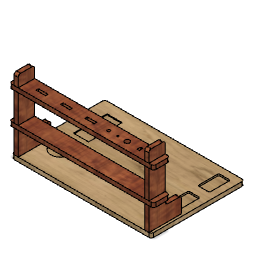
Soldering deskk 18mm v4 (Autodesk Fusion 360 design; units mm, degrees)
Autodesk Fusion 360 part; units mm, degrees
sketch "Limits" plane through (0, 0, 0) normal (0, 1, 0) x (1, 0, 0) in component "Soldering desk v11"
  line L0 (0, 0) -> (-1200, 0)
  line L1 (-1200, 0) -> (-1200, -1200)
  line L2 (-1200, -1200) -> (0, -1200)
  line L3 (0, -1200) -> (0, 0)
  dimension "d5" = 1200
  dimension "d6" = 1200
  constraint horizontal L0
  constraint vertical L1
  constraint horizontal L2
  constraint vertical L3
  constraint coincident L0.start L3.end
  measures "d5" distance of L0.start L0.end
  measures "d6" distance of L0.start L2.end
sketch "Soldering Base" plane through (0, 0, 0) normal (0, 1, 0) x (1, 0, 0) in component "Soldering desk v11"
  line L0 (0, 0) -> (-600, 0)
  line L1 (-600, 0) -> (-600, -400)
  line L2 (-600, -400) -> (0, -400)
  line L3 (0, -400) -> (0, 0)
  line L4 (-28, -350) -> (-10, -350)
  line L5 (-10, -350) -> (-10, -390)
  line L6 (-10, -390) -> (-28, -390)
  line L7 (-28, -390) -> (-28, -350)
  line L8 (-28, -350) -> (-10, -390) construction
  line L9 (-10, -350) -> (-28, -390) construction
  line L10 (-28, -320) -> (-28, -280)
  line L11 (-10, -320) -> (-28, -320)
  line L12 (-10, -280) -> (-10, -320)
  line L13 (-28, -280) -> (-10, -280)
  point P0 (-19, -370)
  dimension "d7" = 600
  dimension "d8" = 400
  dimension "d9" = 18
  dimension "d10" = 40
  dimension "d12" = 10
  dimension "d13" = 10
  dimension "d16" = 0
  dimension "d17" = 70
  constraint horizontal L0
  constraint vertical L1
  constraint horizontal L2
  constraint vertical L3
  constraint coincident L0.start L3.end
  constraint horizontal L4
  constraint perpendicular L4 L5
  constraint parallel L4 L6
  constraint parallel L5 L7
  constraint coincident L8 P0
  constraint coincident L9 P0
  measures "d7" distance of L0.start L0.end
  measures "d8" distance of L0.start L2.end
  measures "d9" distance of L5.end L6.end
  measures "d10" distance of L4.end L5.end
  measures "d12" distance of L3 L5
  measures "d13" distance of L2 L6
extrude "Extrude1" add sketch "Soldering Base" along normal blind 18 makes body 1 in component "Soldering desk v11"
sketch "Stand" plane through (0, 0, 0) normal (1, 0, 0) x (0, 0, -1) in component "Soldering desk v11"
  line L0 (-400, 0) -> (0, 0)
  line L1 (0, 0) -> (0, 18)
  line L2 (0, 18) -> (-400, 18)
  line L3 (-400, 18) -> (-400, 0)
  line L4 (-400, 0) -> (-400, 325)
  line L5 (-400, 325) -> (-330, 325)
  line L6 (-330, 325) -> (-330, 85)
  line L7 (-330, 85) -> (-260, 85)
  line L8 (-400, 0) -> (-260, 0)
  line L9 (-260, 85) -> (-260, 0)
  dimension "d20" = 325
  dimension "d21" = 70
  dimension "d22" = 240
  dimension "d24" = 140
  constraint coincident L0.start L3.end
  constraint perpendicular L0 L4
  constraint perpendicular L4 L5
  constraint perpendicular L5 L6
  constraint perpendicular L6 L7
  constraint perpendicular L4 L8
  constraint perpendicular L8 L9
  measures "d20" distance of L0.start L4.end
  measures "d21" distance of L4.end L5.end
  measures "d22" distance of L5.end L6.end
  measures "d24" distance of L0.start L8.end
extrude "Extrude2" add sketch "Stand" against normal blind 18 from surface at -10 separate body contours L0 L2 L3 L4 L8 L9 | L2 L4 L5 L6 L7 L9 makes body 2 in component "Soldering desk v11"
combine "Combine1" operation cut target body 2 tool bodies 1 keep tools in component "Soldering desk v11"
sketch "Slots" plane through (-10, 0, 0) normal (1, 0, 0) x (0, 0, -1) in component "Soldering desk v11"
  line L0 (-400, 18) -> (-390, 18)
  line L1 (-390, 18) -> (-390, 0)
  line L2 (-390, 0) -> (-350, 0)
  line L3 (-350, 0) -> (-350, 18)
  line L4 (-350, 18) -> (-320, 18)
  line L5 (-320, 18) -> (-320, 0)
  line L6 (-320, 0) -> (-280, 0)
  line L7 (-280, 0) -> (-280, 18)
  line L8 (-280, 18) -> (-260, 18)
  line L9 (-260, 18) -> (-260, 85)
  line L10 (-260, 85) -> (-330, 85)
  line L11 (-330, 85) -> (-330, 325)
  line L12 (-330, 325) -> (-400, 325)
  line L13 (-400, 325) -> (-400, 18)
  line L14 (-400, 276) -> (-360, 276)
  line L15 (-360, 276) -> (-360, 258)
  line L16 (-360, 258) -> (-400, 258)
  line L17 (-400, 258) -> (-400, 276)
  line L18 (-400, 136) -> (-360, 136)
  line L19 (-360, 136) -> (-360, 118)
  line L20 (-360, 118) -> (-400, 118)
  line L21 (-400, 118) -> (-400, 136)
  dimension "d28" = 40
  dimension "d29" = 18
  dimension "d30" = 240
  dimension "d31" = 40
  dimension "d32" = 18
  dimension "d33" = 100
  constraint horizontal L14
  constraint vertical L15
  constraint horizontal L16
  constraint vertical L17
  constraint coincident L13 L14.start
  constraint horizontal L18
  constraint vertical L19
  constraint horizontal L20
  constraint vertical L21
  constraint coincident L13 L18.start
  measures "d28" distance of L14.start L14.end
  measures "d29" distance of L14.start L16.end
  measures "d30" distance of L0 L16
  measures "d31" distance of L18.start L18.end
  measures "d32" distance of L18.start L20.end
  measures "d33" distance of L0 L20
extrude "Extrude3" cut sketch "Slots" against normal blind 18 contours L13 L18 L19 L20 L21 | L13 L14 L15 L16 L17 bodies 2 in component "Soldering desk v11"
extrude "Extrude4" add 1 faces at (-28, 73.6667, 373.3333) along direction (1, 0, 0) blind 18 from surface at -562 on bodies 2 bodies 2 makes body 3 in component "Soldering desk v11"
combine "Combine3" operation cut target body 1 tool bodies 3 keep tools in component "Soldering desk v11"
sketch "Soldering shelves" plane through (0, 0, 400) normal (0, 0, 1) x (1, 0, 0) in component "Soldering desk v11"
  line L0 (-590, 118) -> (-590, 18)
  line L1 (-590, 18) -> (-572, 18)
  line L2 (-572, 18) -> (-572, 118)
  line L3 (-572, 118) -> (-590, 118)
  line L4 (-610, 117.9997) -> (10, 117.9997)
  line L5 (10, 117.9997) -> (10, 135.9997)
  line L6 (10, 135.9997) -> (-610, 135.9997)
  line L7 (-610, 135.9997) -> (-610, 117.9997)
  line L8 (-610, 257.9997) -> (10, 257.9997)
  line L9 (10, 257.9997) -> (10, 275.9997)
  line L10 (10, 275.9997) -> (-610, 275.9997)
  line L11 (-610, 275.9997) -> (-610, 257.9997)
  dimension "d41" = 620
  dimension "d42" = 18
  dimension "d43" = 620
  dimension "d44" = 18
  constraint horizontal L4
  constraint vertical L5
  constraint horizontal L6
  constraint vertical L7
  constraint horizontal L8
  constraint vertical L9
  constraint horizontal L10
  constraint vertical L11
  measures "d41" distance of L4.start L4.end
  measures "d42" distance of L4.start L6.end
  measures "d43" distance of L8.start L8.end
  measures "d44" distance of L8.start L10.end
extrude "Extrude5" add sketch "Soldering shelves" against normal blind 70 separate body contours L3 L4 L5 L6 L7 | L8 L9 L10 L11 makes body 4 at (-196.6667, 275.9997, 376.6667) makes body 5 at (-196.6667, 135.9997, 376.6667) in component "Soldering desk v11"
combine "Combine4" operation cut target body 5 tool bodies 3 keep tools in component "Soldering desk v11"
combine "Combine5" operation cut target body 5 tool bodies 2 keep tools in component "Soldering desk v11"
combine "Combine6" operation cut target body 4 tool bodies 2 keep tools in component "Soldering desk v11"
combine "Combine7" operation cut target body 4 tool bodies 3 keep tools in component "Soldering desk v11"
sketch "Holes for solder" plane through (0, 18, 0) normal (0, 1, 0) x (-1, 0, 0) in component "Soldering desk v11"
  line L0 (590, 280) -> (572, 280)
  line L1 (572, 280) -> (572, 320)
  line L2 (572, 320) -> (590, 320)
  line L3 (590, 320) -> (590, 280)
  line L4 (590, 350) -> (572, 350)
  line L5 (572, 350) -> (572, 390)
  line L6 (572, 390) -> (590, 390)
  line L7 (590, 390) -> (590, 350)
  line L8 (600, 400) -> (0, 400)
  line L9 (0, 400) -> (0, 0)
  line L10 (0, 0) -> (600, 0)
  line L11 (600, 0) -> (600, 400)
  line L12 (28, 320) -> (28, 280)
  line L13 (28, 280) -> (10, 280)
  line L14 (10, 280) -> (10, 320)
  line L15 (10, 320) -> (28, 320)
  line L16 (10, 390) -> (28, 390)
  line L17 (28, 390) -> (28, 350)
  line L18 (28, 350) -> (10, 350)
  line L19 (10, 350) -> (10, 390)
  circle A0 centre (510, 280) radius 41.5
  line L20 (542.5, 192) -> (477.5, 192)
  line L21 (477.5, 192) -> (477.5, 48)
  line L22 (477.5, 48) -> (542.5, 48)
  line L23 (542.5, 48) -> (542.5, 192)
  line L24 (542.5, 192) -> (477.5, 48) construction
  line L25 (477.5, 192) -> (542.5, 48) construction
  line L26 (30, 250) -> (80, 250)
  line L27 (80, 250) -> (80, 160)
  line L28 (80, 160) -> (30, 160)
  line L29 (30, 160) -> (30, 250)
  line L30 (30, 120) -> (80, 120)
  line L31 (80, 120) -> (80, 30)
  line L32 (80, 30) -> (30, 30)
  line L33 (30, 30) -> (30, 120)
  point P0 (510, 120)
  dimension "d49" = 83
  dimension "d50" = 65
  dimension "d51" = 144
  dimension "d54" = 0
  dimension "d55" = -130
  dimension "d82" = 50
  dimension "d83" = 90
  constraint horizontal L20
  constraint perpendicular L20 L21
  constraint parallel L20 L22
  constraint parallel L21 L23
  constraint coincident L24 P0
  constraint coincident L25 P0
  constraint horizontal L26
  constraint vertical L27
  constraint horizontal L28
  constraint vertical L29
  measures "d49" diameter of A0
  measures "d50" distance of L21.end L22.end
  measures "d51" distance of L20.end L21.end
  measures "d82" distance of L30.start L30.end
  measures "d83" distance of L30.end L31.end
extrude "Extrude8" cut sketch "Holes for solder" against normal blind 7 contours L26 L27 L28 L29 | L30 L31 L32 L33 bodies 1 in component "Soldering desk v11"
extrude "Extrude6" cut sketch "Holes for solder" against normal blind 4 contours A0 | L20 L21 L22 L23 bodies 1 in component "Soldering desk v11"
sketch "Holes for tools" plane through (0, 275.9997, 0) normal (0, 1, 0) x (-1, 0, 0) in component "Soldering desk v11"
  line L0 (610, 400) -> (-10, 400)
  line L1 (-10, 400) -> (-10, 330)
  line L2 (-10, 330) -> (10, 330)
  line L3 (10, 330) -> (10, 360)
  line L4 (10, 360) -> (28, 360)
  line L5 (28, 360) -> (28, 330)
  line L6 (590, 330) -> (610, 330)
  line L7 (610, 330) -> (610, 400)
  line L8 (484, 359.75) -> (525, 359.75)
  line L9 (525, 359.75) -> (525, 370.25)
  line L10 (525, 370.25) -> (484, 370.25)
  line L11 (484, 370.25) -> (484, 359.75)
  line L12 (484, 359.75) -> (525, 370.25) construction
  line L13 (525, 359.75) -> (484, 370.25) construction
  line L14 (380, 359.85) -> (420, 359.85)
  line L15 (420, 359.85) -> (420, 370.15)
  line L16 (420, 370.15) -> (380, 370.15)
  line L17 (380, 370.15) -> (380, 359.85)
  line L18 (380, 359.85) -> (420, 370.15) construction
  line L19 (420, 359.85) -> (380, 370.15) construction
  line L20 (315, 359.85) -> (275, 359.85)
  line L21 (275, 359.85) -> (275, 370.15)
  line L22 (275, 370.15) -> (315, 370.15)
  line L23 (315, 370.15) -> (315, 359.85)
  line L24 (315, 359.85) -> (275, 370.15) construction
  line L25 (275, 359.85) -> (315, 370.15) construction
  circle A0 centre (218, 365) radius 6.2
  circle A1 centre (178, 365) radius 3.5
  circle A2 centre (138, 365) radius 10.75
  line L26 (88, 372.4) -> (78, 372.4)
  line L27 (78, 372.4) -> (78, 357.6)
  line L28 (78, 357.6) -> (88, 357.6)
  line L29 (88, 357.6) -> (88, 372.4)
  line L30 (88, 372.4) -> (78, 357.6) construction
  line L31 (78, 372.4) -> (88, 357.6) construction
  line L32 (28, 330) -> (572, 330)
  line L33 (572, 330) -> (572, 360)
  line L34 (572, 360) -> (590, 360)
  line L35 (590, 360) -> (590, 330)
  point P0 (504.5, 365)
  point P1 (400, 365)
  point P2 (295, 365)
  point P3 (83, 365)
  dimension "d58" = 41
  dimension "d59" = 10.5
  dimension "d61" = 40
  dimension "d62" = 10.3
  dimension "d64" = 40
  dimension "d65" = 10.3
  dimension "d67" = 12.4
  dimension "d68" = 7
  dimension "d69" = 21.5
  dimension "d70" = 10
  dimension "d71" = 14.8
  dimension "d72" = 50
  dimension "d73" = 110
  dimension "d74" = 150
  dimension "d75" = 190
  constraint horizontal L8
  constraint perpendicular L8 L9
  constraint parallel L8 L10
  constraint parallel L9 L11
  constraint coincident L12 P0
  constraint coincident L13 P0
  constraint horizontal L14
  constraint perpendicular L14 L15
  constraint parallel L14 L16
  constraint parallel L15 L17
  constraint coincident L18 P1
  constraint coincident L19 P1
  constraint horizontal L20
  constraint perpendicular L20 L21
  constraint parallel L20 L22
  constraint parallel L21 L23
  constraint coincident L24 P2
  constraint coincident L25 P2
  constraint horizontal L26
  constraint perpendicular L26 L27
  constraint parallel L26 L28
  constraint parallel L27 L29
  constraint coincident L30 P3
  constraint coincident L31 P3
  measures "d58" distance of L9.end L10.end
  measures "d59" distance of L8.end L9.end
  measures "d61" distance of L15.end L16.end
  measures "d62" distance of L14.end L15.end
  measures "d64" distance of L21.end L22.end
  measures "d65" distance of L20.end L21.end
  measures "d67" diameter of A0
  measures "d68" diameter of A1
  measures "d69" diameter of A2
  measures "d70" distance of L27.end L28.end
  measures "d71" distance of L26.end L27.end
  measures "d72" distance of L5 L27
  measures "d73" distance of L5 A2.centre
  measures "d74" distance of L5 A1.centre
  measures "d75" distance of L5 A0.centre
extrude "Extrude7" cut sketch "Holes for tools" against normal blind 18 contours L8 L9 L10 L11 | L14 L15 L16 L17 | L20 L21 L22 L23 | A0 | A1 | A2 | L26 L27 L28 L29 bodies 4 in component "Soldering desk v11"
fillet "Fillet1" radius 10 20 edges at (-600, 9, 0) (-600, 9, 400) (0, 9, 400) (0, 9, 0) (-19, 85, 260) (-19, 85, 330) (-19, 325, 330) (-19, 325, 400) (-581, 325, 400) (-581, 325, 330) (-581, 85, 330) (-581, 85, 260) (-610, 266.9997, 330) (-610, 266.9997, 400) (10, 266.9997, 400) (10, 266.9997, 330) (10, 126.9997, 330) (-610, 126.9997, 330) (-610, 126.9997, 400) (10, 126.9997, 400) on bodies 1 2 3 4 5 in component "Soldering desk v11"
fillet "Fillet3" radius 6 8 edges at (-30, 14.5, 250) (-30, 14.5, 120) (-30, 14.5, 160) (-30, 14.5, 30) (-80, 14.5, 30) (-80, 14.5, 160) (-80, 14.5, 250) (-80, 14.5, 120) on bodies 1 in component "Soldering desk v11"
sketch "Soldering Base dxf" plane through (0, 18, 0) normal (0, 1, 0) x (-1, 0, 0) in component "Soldering desk v11"
  line L0 (477.5, 192) -> (542.5, 192)
  line L1 (542.5, 192) -> (542.5, 48)
  line L2 (542.5, 48) -> (477.5, 48)
  line L3 (477.5, 48) -> (477.5, 192)
  circle A0 centre (510, 280) radius 41.5
  line L4 (590, 280) -> (572, 280)
  line L5 (572, 280) -> (572, 320)
  line L6 (572, 320) -> (590, 320)
  line L7 (590, 320) -> (590, 280)
  line L8 (590, 350) -> (572, 350)
  line L9 (572, 350) -> (572, 390)
  line L10 (572, 390) -> (590, 390)
  line L11 (590, 390) -> (590, 350)
  arc A1 (0, 10) -> (10, 0) centre (10, 10) ccw
  line L12 (10, 0) -> (590, 0)
  arc A2 (590, 0) -> (600, 10) centre (590, 10) ccw
  line L13 (600, 10) -> (600, 390)
  arc A3 (600, 390) -> (590, 400) centre (590, 390) ccw
  line L14 (590, 400) -> (10, 400)
  arc A4 (10, 400) -> (0, 390) centre (10, 390) ccw
  line L15 (0, 390) -> (0, 10)
  line L16 (28, 320) -> (28, 280)
  line L17 (28, 280) -> (10, 280)
  line L18 (10, 280) -> (10, 320)
  line L19 (10, 320) -> (28, 320)
  line L20 (10, 390) -> (28, 390)
  line L21 (28, 390) -> (28, 350)
  line L22 (28, 350) -> (10, 350)
  line L23 (10, 350) -> (10, 390)
  line L24 (80, 244) -> (80, 166)
  line L25 (74, 160) -> (36, 160)
  line L26 (30, 166) -> (30, 244)
  line L27 (36, 250) -> (74, 250)
  line L28 (80, 114) -> (80, 36)
  line L29 (74, 30) -> (36, 30)
  line L30 (30, 36) -> (30, 114)
  line L31 (36, 120) -> (74, 120)
  arc A5 (74, 160) -> (80, 166) centre (74, 166) ccw
  arc A6 (30, 166) -> (36, 160) centre (36, 166) ccw
  arc A7 (36, 250) -> (30, 244) centre (36, 244) ccw
  arc A8 (80, 244) -> (74, 250) centre (74, 244) ccw
  arc A9 (74, 30) -> (80, 36) centre (74, 36) ccw
  arc A10 (30, 36) -> (36, 30) centre (36, 36) ccw
  arc A11 (36, 120) -> (30, 114) centre (36, 114) ccw
  arc A12 (80, 114) -> (74, 120) centre (74, 114) ccw
sketch "Left Stand dxf" plane through (-10, 0, 0) normal (1, 0, 0) x (0, 0, -1) in component "Soldering desk v11"
  arc A0 (-390, 325) -> (-400, 315) centre (-390, 315) ccw
  line L0 (-400, 315) -> (-400, 276)
  line L1 (-400, 276) -> (-360, 276)
  line L2 (-360, 276) -> (-360, 258)
  line L3 (-360, 258) -> (-400, 258)
  line L4 (-400, 258) -> (-400, 136)
  line L5 (-400, 136) -> (-360, 136)
  line L6 (-360, 136) -> (-360, 118)
  line L7 (-360, 118) -> (-400, 118)
  line L8 (-400, 118) -> (-400, 18)
  line L9 (-400, 18) -> (-390, 18)
  line L10 (-390, 18) -> (-390, 0)
  line L11 (-390, 0) -> (-350, 0)
  line L12 (-350, 0) -> (-350, 18)
  line L13 (-350, 18) -> (-320, 18)
  line L14 (-320, 18) -> (-320, 0)
  line L15 (-320, 0) -> (-280, 0)
  line L16 (-280, 0) -> (-280, 18)
  line L17 (-280, 18) -> (-260, 18)
  line L18 (-260, 18) -> (-260, 75)
  arc A1 (-260, 75) -> (-270, 85) centre (-270, 75) ccw
  line L19 (-270, 85) -> (-320, 85)
  arc A2 (-330, 95) -> (-320, 85) centre (-320, 95) ccw
  line L20 (-330, 95) -> (-330, 315)
  arc A3 (-330, 315) -> (-340, 325) centre (-340, 315) ccw
  line L21 (-340, 325) -> (-390, 325)
sketch "Right Stand dxf" plane through (-590, 0, 0) normal (-1, 0, 0) x (0, 0, 1) in component "Soldering desk v11"
  arc A0 (270, 85) -> (260, 75) centre (270, 75) ccw
  line L0 (260, 75) -> (260, 18)
  line L1 (260, 18) -> (280, 18)
  line L2 (280, 18) -> (280, 0)
  line L3 (280, 0) -> (320, 0)
  line L4 (320, 0) -> (320, 18)
  line L5 (320, 18) -> (350, 18)
  line L6 (350, 18) -> (350, 0)
  line L7 (350, 0) -> (390, 0)
  line L8 (390, 0) -> (390, 18)
  line L9 (390, 18) -> (400, 18)
  line L10 (400, 18) -> (400, 118)
  line L11 (400, 118) -> (360, 118)
  line L12 (360, 118) -> (360, 136)
  line L13 (360, 136) -> (400, 136)
  line L14 (400, 136) -> (400, 258)
  line L15 (400, 258) -> (360, 258)
  line L16 (360, 258) -> (360, 276)
  line L17 (360, 276) -> (400, 276)
  line L18 (400, 276) -> (400, 315)
  arc A1 (400, 315) -> (390, 325) centre (390, 315) ccw
  line L19 (390, 325) -> (340, 325)
  arc A2 (340, 325) -> (330, 315) centre (340, 315) ccw
  line L20 (330, 315) -> (330, 95)
  arc A3 (320, 85) -> (330, 95) centre (320, 95) ccw
  line L21 (320, 85) -> (270, 85)
sketch "Tools shelf dxf" plane through (0, 275.9997, 0) normal (0, 1, 0) x (-1, 0, 0) in component "Soldering desk v11"
  arc A0 (-10, 340) -> (0, 330) centre (0, 340) ccw
  line L0 (0, 330) -> (10, 330)
  line L1 (10, 330) -> (10, 360)
  line L2 (10, 360) -> (28, 360)
  line L3 (28, 360) -> (28, 330)
  line L4 (28, 330) -> (572, 330)
  line L5 (572, 330) -> (572, 360)
  line L6 (572, 360) -> (590, 360)
  line L7 (590, 360) -> (590, 330)
  arc A1 (600, 330) -> (610, 340) centre (600, 340) ccw
  line L8 (610, 340) -> (610, 390)
  arc A2 (610, 390) -> (600, 400) centre (600, 390) ccw
  line L9 (600, 400) -> (0, 400)
  arc A3 (0, 400) -> (-10, 390) centre (0, 390) ccw
  line L10 (-10, 390) -> (-10, 340)
  line L11 (525, 359.75) -> (484, 359.75)
  line L12 (484, 359.75) -> (484, 370.25)
  line L13 (484, 370.25) -> (525, 370.25)
  line L14 (525, 370.25) -> (525, 359.75)
  circle A4 centre (178, 365) radius 3.5
  circle A5 centre (138, 365) radius 10.75
  line L15 (420, 359.85) -> (380, 359.85)
  line L16 (380, 359.85) -> (380, 370.15)
  line L17 (380, 370.15) -> (420, 370.15)
  line L18 (420, 370.15) -> (420, 359.85)
  circle A6 centre (218, 365) radius 6.2
  line L19 (78, 372.4) -> (88, 372.4)
  line L20 (88, 372.4) -> (88, 357.6)
  line L21 (88, 357.6) -> (78, 357.6)
  line L22 (78, 357.6) -> (78, 372.4)
  line L23 (275, 359.85) -> (275, 370.15)
  line L24 (275, 370.15) -> (315, 370.15)
  line L25 (315, 370.15) -> (315, 359.85)
  line L26 (315, 359.85) -> (275, 359.85)
  line L27 (590, 330) -> (600, 330)
sketch "Storage shelf dxf" plane through (0, 135.9997, 0) normal (0, 1, 0) x (-1, 0, 0) in component "Soldering desk v11"
  arc A0 (0, 400) -> (-10, 390) centre (0, 390) ccw
  line L0 (-10, 390) -> (-10, 340)
  arc A1 (-10, 340) -> (0, 330) centre (0, 340) ccw
  line L1 (0, 330) -> (10, 330)
  line L2 (10, 330) -> (10, 360)
  line L3 (10, 360) -> (28, 360)
  line L4 (28, 360) -> (28, 330)
  line L5 (572, 330) -> (572, 360)
  line L6 (572, 360) -> (590, 360)
  line L7 (590, 360) -> (590, 330)
  arc A2 (600, 330) -> (610, 340) centre (600, 340) ccw
  line L8 (610, 340) -> (610, 390)
  arc A3 (610, 390) -> (600, 400) centre (600, 390) ccw
  line L9 (600, 400) -> (0, 400)
  line L10 (590, 330) -> (600, 330)
  line L11 (28, 330) -> (572, 330)
component "Soldering desk v11" placed x (1, 0, 0) y (0, 1, 0) z (0, 0, 1) at (0, 0, 0)
equation "Length = 600 mm"
equation "Height = 325 mm"
equation "breadth = 400 mm"
equation "thickness = 18 mm"
equation "d7 = Length"
equation "d8 = breadth"
equation "d9 = thickness"
equation "d10 = HoleStandB"
equation "d12 = gapStand"
equation "d13 = gapStand"
equation "d18 = thickness"
equation "d20 = Height"
equation "d21 = TopStandB"
equation "d22 = MidStandH"
equation "d24 = BottomStandB"
equation "d26 = -thickness"
equation "d28 = slotL"
equation "d29 = thickness"
equation "d30 = GapslotS2H"
equation "d31 = slotL"
equation "d32 = thickness"
equation "d33 = GapslotS1H"
equation "d34 = -thickness"
equation "d37 = -thickness"
equation "d41 = shelfL"
equation "d42 = thickness"
equation "d43 = shelfL"
equation "d44 = thickness"
equation "d45 = -shelfB"
equation "d49 = TipCleanerD"
equation "d50 = IronHolderB"
equation "d51 = IronStandL"
equation "d56 = -C2Hole"
equation "d58 = wirestripperB"
equation "d59 = wireStripperT"
equation "d61 = cutpilerB"
equation "d62 = cutpilerT"
equation "d64 = cutpilerB"
equation "d65 = cutpilerT"
equation "d67 = D1"
equation "d68 = D2"
equation "d69 = D3"
equation "d70 = pcbHolderB"
equation "d71 = pcbHolderT"
equation "d76 = -thickness"
equation "d79 = fillet"
equation "d82 = containerB"
equation "d83 = containerL"
equation "HoleStandB = 40 mm"
equation "gapStand = 10 mm"
equation "TopStandB = 70 mm"
equation "BottomStandB = 140 mm"
equation "MidStandH = 240 mm"
equation "slotL = 40 mm"
equation "GapslotS1H = 100 mm"
equation "GapslotS2H = 240 mm"
equation "shelfL = 620 mm"
equation "containerL = 90 mm"
equation "containerB = 50 mm"
equation "TipCleanerD = 83 mm"
equation "IronStandL = 144 mm"
equation "IronHolderB = 65 mm"
equation "cutpilerB = 40 mm"
equation "cutpilerT = 10.3 mm"
equation "wirestripperB = 41 mm"
equation "wireStripperT = 10.5 mm"
equation "D1 = 12.4 mm"
equation "D2 = 7 mm"
equation "D3 = 21.5 mm"
equation "pcbHolderB = 10 mm"
equation "pcbHolderT = 14.8 mm"
equation "fillet = 10 mm"
equation "containerFillet = 6 mm"
equation "ContainerHole = 7 mm"
equation "C2Hole = 4 mm"
equation "d111 = -ContainerHole"
equation "d114 = containerFillet"
equation "shelfB = 70 mm"
named bodies: "Soldering Base", "Left Stand", "Right stand", "Tools shelf", "Storage shelf"
